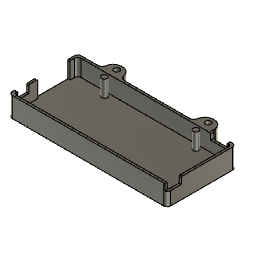
AramBadgeCase (Autodesk Fusion 360 design; units mm, degrees)
Autodesk Fusion 360 part; units mm, degrees
sketch "Sketch1" plane through (0, 0, 0) normal (0, 0, 1) x (1, 0, 0)
  line L0 (69.25, -29) -> (-69.25, -29)
  line L1 (-69.25, -29) -> (-69.25, 29)
  line L2 (-69.25, 29) -> (69.25, 29)
  line L3 (69.25, 29) -> (69.25, -29)
  line L4 (69.25, -29) -> (-69.25, 29) construction
  line L5 (-69.25, -29) -> (69.25, 29) construction
  line L6 (71.25, -31) -> (-71.25, -31)
  line L7 (-71.25, -31) -> (-71.25, 31)
  line L8 (-71.25, 31) -> (71.25, 31)
  line L9 (71.25, 31) -> (71.25, -31)
  line L10 (71.25, -31) -> (-71.25, 31) construction
  line L11 (-71.25, -31) -> (71.25, 31) construction
  dimension "d1" = 138.5
  dimension "d2" = 58
  dimension "d3" = 2
  dimension "d4" = 2
  constraint horizontal L0
  constraint perpendicular L0 L1
  constraint parallel L0 L2
  constraint parallel L1 L3
  constraint coincident L4 origin
  constraint coincident L5 origin
  constraint horizontal L6
  constraint perpendicular L6 L7
  constraint parallel L6 L8
  constraint parallel L7 L9
  constraint coincident L10 origin
  constraint coincident L11 origin
  measures "d1" distance of L1.end L2.end
  measures "d2" distance of L0.end L1.end
  measures "d3" distance of L1 L7
  measures "d4" distance of L2 L8
extrude "Extrude1" add sketch "Sketch1" along normal blind 15 makes body 1
sketch "Sketch3" plane through (0, 0, 15) normal (0, 0, 1) x (-1, 0, 0)
  line L0 (69.25, -29) -> (-69.25, -29)
  line L1 (-69.25, -29) -> (-69.25, 29)
  line L2 (-69.25, 29) -> (69.25, 29)
  line L3 (69.25, 29) -> (69.25, -29)
  line L4 (71.25, 31) -> (-71.25, 31)
  line L5 (-71.25, 31) -> (-71.25, -31)
  line L6 (-71.25, -31) -> (71.25, -31)
  line L7 (71.25, -31) -> (71.25, 31)
  line L8 (-65.25, -29) -> (-65.25, -31)
  line L9 (-50.25, -31) -> (-50.25, -29)
  line L10 (-69.25, 18) -> (-71.25, 18)
  line L11 (-71.25, 18) -> (-71.25, 31)
  line L12 (-71.25, 31) -> (-69.25, 31)
  line L13 (-69.25, 31) -> (-69.25, 18)
  line L14 (71.25, 15) -> (69.25, 15)
  line L15 (69.25, 25) -> (71.25, 25)
  dimension "d13" = 21
  dimension "d14" = 6
  dimension "d19" = 13
  dimension "d22" = 6
  dimension "d23" = 16
  constraint vertical L8
  constraint vertical L9
  constraint coincident L6 L8.end
  constraint coincident L0 L9.end
  constraint horizontal L10
  constraint vertical L11
  constraint horizontal L12
  constraint vertical L13
  constraint coincident L4.end L5.start
  constraint coincident L1 L10.start
  constraint horizontal L14
  constraint horizontal L15
  constraint coincident L3 L15.start
  constraint coincident L7 L14.start
  measures "d13" distance of L5.end L9
  measures "d14" distance of L5 L8
  measures "d19" distance of L10 L12
  measures "d22" distance of L4 L15.start
  measures "d23" distance of L4 L14.start
extrude "Extrude5" cut sketch "Sketch3" against normal blind 7 contours L3 L7 L14 L15 bodies 1
extrude "Extrude3" cut sketch "Sketch3" against normal blind 5.5 contours L0 L6 L8 L9 bodies 1
sketch "Sketch2" plane through (0, 0, 0) normal (0, 0, -1) x (1, 0, 0)
  line L0 (-71.25, 31) -> (-71.25, -31)
  line L1 (-71.25, -31) -> (71.25, -31)
  line L2 (71.25, -31) -> (71.25, 31)
  line L3 (71.25, 31) -> (-71.25, 31)
  line L4 (-69.25, -29) -> (-69.25, 29)
  line L5 (-69.25, 29) -> (69.25, 29)
  line L6 (69.25, 29) -> (69.25, -29)
  line L7 (69.25, -29) -> (-69.25, -29)
  circle A0 centre (41.25, -25) radius 2.5
  line L8 (-69.25, -29) -> (69.25, -29)
  line L9 (69.25, -29) -> (69.25, 29)
  dimension "d32" = 5
  dimension "d33" = 4
  dimension "d34" = 28
  measures "d32" diameter of A0
  measures "d33" distance of A0.centre L8
  measures "d34" distance of A0.centre L9
extrude "Extrude6" add sketch "Sketch2" against normal up to surface (15 mm away) separate body contours A0 makes body 2
extrude "Extrude2" add sketch "Sketch2" along normal blind 3 contours L0 L1 L2 L3 | L4 L5 L6 L7 L8 L9 | A0 bodies 1
extrude "Extrude4" cut sketch "Sketch3" against normal blind 6 contours L1 L4 L5 L10 L11 L12 L13 bodies 1
fillet "Fillet4" radius 3 4 edges at (71.25, -31, 3) (71.25, 31, 6) (-71.25, -31, 6) (-71.25, 31, 6) on bodies 1
fillet "Fillet5" radius 3 4 edges at (69.25, 29, 7.5) (-69.25, 29, 7.5) (-69.25, -29, 7.5) (69.25, -29, 4.5) on bodies 1
fillet "Fillet6" radius 1 5 edges at (-70.25, -15, 15) (-70.25, -25, 15) (65.25, 30, 15) (50.25, 30, 15) (70.25, -18, 15) on bodies 1
mirror "Mirror1" about plane through (0, 0, 0) normal (1, 0, 0) of bodies 2 makes body 3
sketch "Sketch4" plane through (0, 0, 15) normal (0, 0, 1) x (-1, 0, 0)
  line L0 (-49.25, -29) -> (-49.25, -31)
  line L1 (-49.25, -31) -> (68.25, -31)
  arc A0 (68.25, -31) -> (71.25, -28) centre (68.25, -28) ccw
  line L2 (71.25, -28) -> (71.25, 14)
  line L3 (71.25, 14) -> (69.25, 14)
  line L4 (69.25, 14) -> (69.25, -26)
  arc A1 (66.25, -29) -> (69.25, -26) centre (66.25, -26) ccw
  line L5 (66.25, -29) -> (-49.25, -29)
  line L6 (71.25, -22) -> (69.25, -22)
  line L7 (69.25, -22) -> (69.25, 7)
  line L8 (69.25, 7) -> (71.25, 7)
  line L9 (71.25, 7) -> (71.25, -22)
  line L10 (71.25, -31) -> (-71.25, -31)
  dimension "d39" = 9
  dimension "d40" = 38
  constraint horizontal L6
  constraint vertical L7
  constraint horizontal L8
  constraint vertical L9
  constraint coincident L4 L7.end
  constraint coincident L2 L6.start
  measures "d39" distance of L6 L10
  measures "d40" distance of L8 L10
extrude "Extrude7" cut sketch "Sketch4" against normal up to surface (15 mm away) contours L2 L4 L6 L7 L8 L9 bodies 1
fillet "Fillet7" radius 1 2 edges at (-70.25, 22, 15) (-70.25, -7, 15) on bodies 1
sketch "Sketch6" plane through (0, 31, 0) normal (0, 1, 0) x (-1, 0, 0)
  arc A0 (-49.25, 15) -> (-50.25, 14) centre (-49.25, 14) ccw
  line L0 (-50.25, 14) -> (-50.25, 9.5)
  line L1 (-50.25, 9.5) -> (-65.25, 9.5)
  line L2 (-65.25, 9.5) -> (-65.25, 14)
  arc A1 (-65.25, 14) -> (-66.25, 15) centre (-66.25, 14) ccw
  line L3 (-66.25, 15) -> (-68.25, 15)
  line L4 (-68.25, 15) -> (-68.25, -3)
  line L5 (-68.25, -3) -> (68.25, -3)
  line L6 (68.25, -3) -> (68.25, 15)
  line L7 (68.25, 15) -> (-49.25, 15)
  line L8 (-33.25, 15) -> (-49.25, 15)
  line L9 (-49.25, 15) -> (-49.25, -3)
  line L10 (-49.25, -3) -> (-33.25, -3)
  line L11 (-33.25, -3) -> (-33.25, 15)
  dimension "d47" = 19
  dimension "d48" = 16
  constraint horizontal L8
  constraint vertical L9
  constraint horizontal L10
  constraint vertical L11
  constraint coincident L5 L9.end
  constraint coincident L7 L8.start
  measures "d47" distance of L4 L9
  measures "d48" distance of L9 L11
extrude "Extrude9" add sketch "Sketch6" along normal blind 10 contours L5 L7 L8 L9 L10 L11 bodies 1
sketch "Sketch7" plane through (0, 0, 15) normal (0, 0, 1) x (-1, 0, 0)
  line L0 (71.25, -23) -> (69.25, -23)
  line L1 (69.25, -23) -> (69.25, -26)
  arc A0 (66.25, -29) -> (69.25, -26) centre (66.25, -26) ccw
  line L2 (66.25, -29) -> (-49.25, -29)
  line L3 (-49.25, -29) -> (-49.25, -31)
  line L4 (-49.25, -31) -> (-49.25, -41)
  line L5 (-49.25, -41) -> (-33.25, -41)
  line L6 (-33.25, -41) -> (-33.25, -31)
  line L7 (-33.25, -31) -> (68.25, -31)
  arc A1 (68.25, -31) -> (71.25, -28) centre (68.25, -28) ccw
  line L8 (71.25, -28) -> (71.25, -23)
  circle A2 centre (-41.25, -36) radius 2.5
  dimension "d51" = 5
  dimension "d52" = 8
  dimension "d53" = 5
  measures "d51" diameter of A2
  measures "d52" distance of L4 A2.centre
  measures "d53" distance of L5 A2.centre
extrude "Extrude10" cut sketch "Sketch7" against normal up to surface (18 mm away) contours A2 bodies 1
fillet "Fillet8" radius 7.5 2 edges at (49.25, 41, 6) (33.25, 41, 6) on bodies 1
mirror "Mirror2" about plane through (0, 0, 0) normal (1, 0, 0) of "Extrude9", "Extrude10", "Fillet8"
sketch "Sketch8" plane through (0, 0, -3) normal (0, 0, -1) x (1, 0, 0)
  circle A0 centre (-41.25, -36) radius 2.5
  arc A1 (-40.75, -41) -> (-33.25, -33.5) centre (-40.75, -33.5) ccw
  line L0 (-33.25, -33.5) -> (-33.25, -31)
  line L1 (-33.25, -31) -> (33.25, -31)
  line L2 (33.25, -31) -> (33.25, -33.5)
  arc A2 (33.25, -33.5) -> (40.75, -41) centre (40.75, -33.5) ccw
  line L3 (40.75, -41) -> (41.75, -41)
  arc A3 (41.75, -41) -> (49.25, -33.5) centre (41.75, -33.5) ccw
  line L4 (49.25, -33.5) -> (49.25, -31)
  line L5 (49.25, -31) -> (68.25, -31)
  arc A4 (68.25, -31) -> (71.25, -28) centre (68.25, -28) ccw
  line L6 (71.25, -28) -> (71.25, 28)
  arc A5 (71.25, 28) -> (68.25, 31) centre (68.25, 28) ccw
  line L7 (68.25, 31) -> (-68.25, 31)
  arc A6 (-68.25, 31) -> (-71.25, 28) centre (-68.25, 28) ccw
  line L8 (-71.25, 28) -> (-71.25, -28)
  arc A7 (-71.25, -28) -> (-68.25, -31) centre (-68.25, -28) ccw
  line L9 (-68.25, -31) -> (-49.25, -31)
  line L10 (-49.25, -31) -> (-49.25, -33.5)
  arc A8 (-49.25, -33.5) -> (-41.75, -41) centre (-41.75, -33.5) ccw
  line L11 (-41.75, -41) -> (-40.75, -41)
  circle A9 centre (41.25, -36) radius 2.5
  line L12 (-0.7094, -15.2047) -> (66.5141, -15.2047)
  line L13 (66.5141, -15.2047) -> (66.5141, 0.5508)
  line L14 (66.5141, 0.5508) -> (66.5141, 16.3063)
  line L15 (66.5141, 16.3063) -> (-0.7094, 16.3063)
  line L16 (-0.7094, 16.3063) -> (-67.9329, 16.3063)
  line L17 (-67.9329, 16.3063) -> (-67.9329, 0.5508)
  line L18 (-67.9329, 0.5508) -> (-67.9329, -15.2047)
  line L19 (-67.9329, -15.2047) -> (-0.7094, -15.2047)
  spline S0 degree 3 poles (-57.2192, 7.9034) (-55.8537, 7.9034) (-56.2739, 5.5926) (-58.1645, 3.4918) knots 0 0 0 0 1 1 1 1
  spline S1 degree 3 poles (-58.1645, 3.4918) (-59.7401, 1.7062) (-59.7401, 1.4961) (-57.9544, -0.4996) knots 0 0 0 0 1 1 1 1
  spline S2 degree 3 poles (-57.9544, -0.4996) (-54.9084, -3.8607) (-57.1141, -4.2809) (-60.5804, -1.0247) knots 0 0 0 0 1 1 1 1
  line L20 (-60.5804, -1.0247) -> (-63.7315, 2.0213)
  line L21 (-63.7315, 2.0213) -> (-60.8955, 4.9624)
  spline S3 degree 3 poles (-60.8955, 4.9624) (-59.3199, 6.5379) (-57.7444, 7.9034) (-57.2192, 7.9034) knots 0 0 0 0 1 1 1 1
  spline S4 degree 3 poles (-52.7026, 7.9034) (-51.5472, 7.9034) (-51.1271, 6.6429) (-51.1271, 2.6515) knots 0 0 0 0 1 1 1 1
  line L22 (-51.1271, 2.6515) -> (-51.1271, -2.6003)
  line L23 (-51.1271, -2.6003) -> (-47.4508, -2.6003)
  line L24 (-47.4508, -2.6003) -> (-43.7745, -2.6003)
  line L25 (-43.7745, -2.6003) -> (-43.7745, 2.6515)
  spline S5 degree 3 poles (-43.7745, 2.6515) (-43.7745, 6.6429) (-43.3543, 7.9034) (-42.1989, 7.9034) knots 0 0 0 0 1 1 1 1
  spline S6 degree 3 poles (-42.1989, 7.9034) (-40.9385, 7.9034) (-40.6234, 6.5379) (-40.6234, 2.1264) knots 0 0 0 0 1 1 1 1
  spline S7 degree 3 poles (-40.6234, 2.1264) (-40.6234, -4.0708) (-41.9889, -5.7514) (-47.4508, -5.7514) knots 0 0 0 0 1 1 1 1
  spline S8 degree 3 poles (-47.4508, -5.7514) (-52.9127, -5.7514) (-54.2782, -4.0708) (-54.2782, 2.1264) knots 0 0 0 0 1 1 1 1
  spline S9 degree 3 poles (-54.2782, 2.1264) (-54.2782, 6.5379) (-53.963, 7.9034) (-52.7026, 7.9034) knots 0 0 0 0 1 1 1 1
  spline S10 degree 3 poles (-37.2622, 6.6429) (-35.5816, 8.3235) (-27.8089, 8.3235) (-26.1283, 6.6429) knots 0 0 0 0 1 1 1 1
  spline S11 degree 3 poles (-26.1283, 6.6429) (-24.4477, 4.9624) (-24.6578, -2.3902) (-26.4434, -6.2766) knots 0 0 0 0 1 1 1 1
  spline S12 degree 3 poles (-26.4434, -6.2766) (-27.3887, -8.3773) (-27.9139, -8.7975) (-27.9139, -7.537) knots 0 0 0 0 1 1 1 1
  spline S13 degree 3 poles (-27.9139, -7.537) (-28.019, -6.1715) (-28.9643, -5.7514) (-31.6953, -5.7514) knots 0 0 0 0 1 1 1 1
  spline S14 degree 3 poles (-31.6953, -5.7514) (-34.4262, -5.7514) (-35.3715, -6.1715) (-35.4766, -7.537) knots 0 0 0 0 1 1 1 1
  spline S15 degree 3 poles (-35.4766, -7.537) (-35.4766, -8.7975) (-36.0018, -8.3773) (-36.9471, -6.2766) knots 0 0 0 0 1 1 1 1
  spline S16 degree 3 poles (-36.9471, -6.2766) (-38.7327, -2.3902) (-38.9428, 4.9624) (-37.2622, 6.6429) knots 0 0 0 0 1 1 1 1
  line L26 (-17.5153, -2.6003) -> (-12.2635, -2.6003)
  line L27 (-12.2635, -2.6003) -> (-12.2635, 1.076)
  line L28 (-12.2635, 1.076) -> (-12.2635, 4.7523)
  line L29 (-12.2635, 4.7523) -> (-17.5153, 4.7523)
  spline S17 degree 3 poles (-17.5153, 4.7523) (-21.5067, 4.7523) (-22.7671, 5.1724) (-22.7671, 6.3278) knots 0 0 0 0 1 1 1 1
  spline S18 degree 3 poles (-22.7671, 6.3278) (-22.7671, 8.3235) (-12.2635, 8.5336) (-10.3728, 6.6429) knots 0 0 0 0 1 1 1 1
  spline S19 degree 3 poles (-10.3728, 6.6429) (-9.6375, 5.9077) (-9.1124, 3.3868) (-9.1124, 0.8659) knots 0 0 0 0 1 1 1 1
  spline S20 degree 3 poles (-9.1124, 0.8659) (-9.1124, -4.491) (-10.898, -5.7514) (-17.9354, -5.7514) knots 0 0 0 0 1 1 1 1
  spline S21 degree 3 poles (-17.9354, -5.7514) (-21.5067, -5.7514) (-22.7671, -5.3312) (-22.7671, -4.1758) knots 0 0 0 0 1 1 1 1
  spline S22 degree 3 poles (-22.7671, -4.1758) (-22.7671, -3.0204) (-21.5067, -2.6003) (-17.5153, -2.6003) knots 0 0 0 0 1 1 1 1
  spline S23 degree 3 poles (-5.4361, 7.9034) (-4.2807, 7.9034) (-3.8605, 6.6429) (-3.8605, 2.6515) knots 0 0 0 0 1 1 1 1
  line L30 (-3.8605, 2.6515) -> (-3.8605, -2.6003)
  line L31 (-3.8605, -2.6003) -> (-0.1842, -2.6003)
  line L32 (-0.1842, -2.6003) -> (3.4921, -2.6003)
  line L33 (3.4921, -2.6003) -> (3.4921, 2.6515)
  spline S24 degree 3 poles (3.4921, 2.6515) (3.4921, 6.6429) (3.9122, 7.9034) (5.0676, 7.9034) knots 0 0 0 0 1 1 1 1
  spline S25 degree 3 poles (5.0676, 7.9034) (6.328, 7.9034) (6.6432, 6.5379) (6.6432, 2.1264) knots 0 0 0 0 1 1 1 1
  spline S26 degree 3 poles (6.6432, 2.1264) (6.6432, -4.0708) (5.2777, -5.7514) (-0.1842, -5.7514) knots 0 0 0 0 1 1 1 1
  spline S27 degree 3 poles (-0.1842, -5.7514) (-5.6461, -5.7514) (-7.0116, -4.0708) (-7.0116, 2.1264) knots 0 0 0 0 1 1 1 1
  spline S28 degree 3 poles (-7.0116, 2.1264) (-7.0116, 6.5379) (-6.6965, 7.9034) (-5.4361, 7.9034) knots 0 0 0 0 1 1 1 1
  spline S29 degree 3 poles (-0.1842, 7.9034) (0.9712, 7.9034) (1.3913, 6.6429) (1.3913, 3.1767) knots 0 0 0 0 1 1 1 1
  spline S30 degree 3 poles (1.3913, 3.1767) (1.3913, -0.2895) (0.9712, -1.5499) (-0.1842, -1.5499) knots 0 0 0 0 1 1 1 1
  spline S31 degree 3 poles (-0.1842, -1.5499) (-1.3396, -1.5499) (-1.7598, -0.2895) (-1.7598, 3.1767) knots 0 0 0 0 1 1 1 1
  spline S32 degree 3 poles (-1.7598, 3.1767) (-1.7598, 6.6429) (-1.3396, 7.9034) (-0.1842, 7.9034) knots 0 0 0 0 1 1 1 1
  spline S33 degree 3 poles (10.3194, 7.9034) (11.2648, 7.9034) (11.895, 6.9581) (11.895, 5.2775) knots 0 0 0 0 1 1 1 1
  spline S34 degree 3 poles (11.895, 5.2775) (11.895, 2.9667) (12.3151, 2.6515) (15.5713, 2.6515) knots 0 0 0 0 1 1 1 1
  spline S35 degree 3 poles (15.5713, 2.6515) (18.8274, 2.6515) (19.2476, 2.9667) (19.2476, 5.2775) knots 0 0 0 0 1 1 1 1
  spline S36 degree 3 poles (19.2476, 5.2775) (19.2476, 6.9581) (19.8778, 7.9034) (20.8231, 7.9034) knots 0 0 0 0 1 1 1 1
  spline S37 degree 3 poles (20.8231, 7.9034) (23.0289, 7.9034) (23.0289, -1.865) (20.7181, -4.0708) knots 0 0 0 0 1 1 1 1
  spline S38 degree 3 poles (20.7181, -4.0708) (18.8274, -5.9615) (13.7857, -6.2766) (10.7396, -4.701) knots 0 0 0 0 1 1 1 1
  spline S39 degree 3 poles (10.7396, -4.701) (9.164, -3.7557) (8.7439, -2.3902) (8.7439, 2.1264) knots 0 0 0 0 1 1 1 1
  spline S40 degree 3 poles (8.7439, 2.1264) (8.7439, 6.5379) (9.059, 7.9034) (10.3194, 7.9034) knots 0 0 0 0 1 1 1 1
  spline S41 degree 3 poles (29.9613, 2.4415) (34.4779, 2.7566) (35.0031, 2.9667) (35.0031, 5.3825) knots 0 0 0 0 1 1 1 1
  spline S42 degree 3 poles (35.0031, 5.3825) (35.0031, 6.9581) (35.6333, 7.9034) (36.5786, 7.9034) knots 0 0 0 0 1 1 1 1
  spline S43 degree 3 poles (36.5786, 7.9034) (37.8391, 7.9034) (38.1542, 6.4329) (38.1542, 1.076) knots 0 0 0 0 1 1 1 1
  line L34 (38.1542, 1.076) -> (38.1542, -5.7514)
  line L35 (38.1542, -5.7514) -> (32.5872, -5.7514)
  spline S44 degree 3 poles (32.5872, -5.7514) (26.285, -5.7514) (24.2893, -4.3859) (24.7095, -0.4996) knots 0 0 0 0 1 1 1 1
  spline S45 degree 3 poles (24.7095, -0.4996) (25.0246, 1.8113) (25.5498, 2.1264) (29.9613, 2.4415) knots 0 0 0 0 1 1 1 1
  spline S46 degree 3 poles (29.2261, 7.9034) (30.0664, 7.9034) (30.8016, 6.9581) (30.8016, 5.8026) knots 0 0 0 0 1 1 1 1
  spline S47 degree 3 poles (30.8016, 5.8026) (30.8016, 4.6472) (30.0664, 3.7019) (29.2261, 3.7019) knots 0 0 0 0 1 1 1 1
  spline S48 degree 3 poles (29.2261, 3.7019) (28.3858, 3.7019) (27.6505, 4.6472) (27.6505, 5.8026) knots 0 0 0 0 1 1 1 1
  spline S49 degree 3 poles (27.6505, 5.8026) (27.6505, 6.9581) (28.3858, 7.9034) (29.2261, 7.9034) knots 0 0 0 0 1 1 1 1
  spline S50 degree 3 poles (41.2002, 7.9034) (41.7254, 7.9034) (42.3557, 6.853) (42.5657, 5.5926) knots 0 0 0 0 1 1 1 1
  spline S51 degree 3 poles (42.5657, 5.5926) (42.7758, 3.5969) (43.6161, 3.0717) (46.7672, 2.8616) knots 0 0 0 0 1 1 1 1
  spline S52 degree 3 poles (46.7672, 2.8616) (50.4435, 2.5465) (50.7586, 2.7566) (50.7586, 5.1724) knots 0 0 0 0 1 1 1 1
  spline S53 degree 3 poles (50.7586, 5.1724) (50.7586, 6.853) (51.3888, 7.9034) (52.3341, 7.9034) knots 0 0 0 0 1 1 1 1
  spline S54 degree 3 poles (52.3341, 7.9034) (54.5399, 7.9034) (54.5399, -1.865) (52.2291, -4.0708) knots 0 0 0 0 1 1 1 1
  spline S55 degree 3 poles (52.2291, -4.0708) (50.3384, -5.9615) (45.2967, -6.2766) (42.2506, -4.701) knots 0 0 0 0 1 1 1 1
  spline S56 degree 3 poles (42.2506, -4.701) (40.6751, -3.7557) (40.2549, -2.3902) (40.2549, 2.1264) knots 0 0 0 0 1 1 1 1
  spline S57 degree 3 poles (40.2549, 2.1264) (40.2549, 5.2775) (40.6751, 7.9034) (41.2002, 7.9034) knots 0 0 0 0 1 1 1 1
  line L36 (58.1112, 0.0256) -> (60.2119, 2.3364)
  line L37 (60.2119, 2.3364) -> (58.1112, 4.2271)
  spline S58 degree 3 poles (58.1112, 4.2271) (56.9558, 5.2775) (56.0104, 6.5379) (56.0104, 7.0631) knots 0 0 0 0 1 1 1 1
  spline S59 degree 3 poles (56.0104, 7.0631) (56.0104, 8.8487) (58.8464, 7.7983) (61.5774, 4.9624) knots 0 0 0 0 1 1 1 1
  line L38 (61.5774, 4.9624) -> (64.4134, 2.0213)
  line L39 (64.4134, 2.0213) -> (61.4723, -0.8147)
  spline S60 degree 3 poles (61.4723, -0.8147) (56.8507, -5.2262) (53.9097, -4.491) (58.1112, 0.0256) knots 0 0 0 0 1 1 1 1
  spline S61 degree 3 poles (-31.6953, -2.6003) (-28.229, -2.6003) (-28.019, -2.3902) (-28.019, 1.076) knots 0 0 0 0 1 1 1 1
  spline S62 degree 3 poles (-28.019, 1.076) (-28.019, 4.5422) (-28.229, 4.7523) (-31.6953, 4.7523) knots 0 0 0 0 1 1 1 1
  spline S63 degree 3 poles (-31.6953, 4.7523) (-35.1615, 4.7523) (-35.3715, 4.5422) (-35.3715, 1.076) knots 0 0 0 0 1 1 1 1
  spline S64 degree 3 poles (-35.3715, 1.076) (-35.3715, -2.3902) (-35.1615, -2.6003) (-31.6953, -2.6003) knots 0 0 0 0 1 1 1 1
  spline S65 degree 3 poles (-33.2708, 0.5508) (-32.7456, 0.5508) (-32.2204, 0.1307) (-32.2204, -0.4996) knots 0 0 0 0 1 1 1 1
  spline S66 degree 3 poles (-32.2204, -0.4996) (-32.2204, -1.0247) (-32.7456, -1.5499) (-33.2708, -1.5499) knots 0 0 0 0 1 1 1 1
  spline S67 degree 3 poles (-33.2708, -1.5499) (-33.901, -1.5499) (-34.3212, -1.0247) (-34.3212, -0.4996) knots 0 0 0 0 1 1 1 1
  spline S68 degree 3 poles (-34.3212, -0.4996) (-34.3212, 0.1307) (-33.901, 0.5508) (-33.2708, 0.5508) knots 0 0 0 0 1 1 1 1
  spline S69 degree 3 poles (-30.1197, 0.5508) (-29.5945, 0.5508) (-29.0693, 0.1307) (-29.0693, -0.4996) knots 0 0 0 0 1 1 1 1
  spline S70 degree 3 poles (-29.0693, -0.4996) (-29.0693, -1.0247) (-29.5945, -1.5499) (-30.1197, -1.5499) knots 0 0 0 0 1 1 1 1
  spline S71 degree 3 poles (-30.1197, -1.5499) (-30.7499, -1.5499) (-31.1701, -1.0247) (-31.1701, -0.4996) knots 0 0 0 0 1 1 1 1
  spline S72 degree 3 poles (-31.1701, -0.4996) (-31.1701, 0.1307) (-30.7499, 0.5508) (-30.1197, 0.5508) knots 0 0 0 0 1 1 1 1
  spline S73 degree 3 poles (15.2562, -2.3902) (17.0418, -2.1801) (18.7224, -1.5499) (18.9325, -0.9197) knots 0 0 0 0 1 1 1 1
  spline S74 degree 3 poles (18.9325, -0.9197) (19.1425, -0.2895) (17.8821, -0.0794) (15.5713, -0.2895) knots 0 0 0 0 1 1 1 1
  spline S75 degree 3 poles (15.5713, -0.2895) (10.9497, -0.8147) (10.6346, -2.8104) (15.2562, -2.3902) knots 0 0 0 0 1 1 1 1
  spline S76 degree 3 poles (31.3268, -2.6003) (33.6376, -2.6003) (35.0031, -2.0751) (35.0031, -1.2348) knots 0 0 0 0 1 1 1 1
  spline S77 degree 3 poles (35.0031, -1.2348) (35.0031, -0.2895) (33.8477, 0.0256) (31.3268, -0.2895) knots 0 0 0 0 1 1 1 1
  spline S78 degree 3 poles (31.3268, -0.2895) (29.3311, -0.4996) (27.6505, -1.1298) (27.6505, -1.655) knots 0 0 0 0 1 1 1 1
  spline S79 degree 3 poles (27.6505, -1.655) (27.6505, -2.1801) (29.3311, -2.6003) (31.3268, -2.6003) knots 0 0 0 0 1 1 1 1
  spline S80 degree 3 poles (46.7672, -2.3902) (48.5528, -2.1801) (50.2334, -1.5499) (50.4435, -0.9197) knots 0 0 0 0 1 1 1 1
  spline S81 degree 3 poles (50.4435, -0.9197) (50.6536, -0.2895) (49.3931, -0.0794) (47.0823, -0.2895) knots 0 0 0 0 1 1 1 1
  spline S82 degree 3 poles (47.0823, -0.2895) (42.4607, -0.8147) (42.1456, -2.8104) (46.7672, -2.3902) knots 0 0 0 0 1 1 1 1
extrude "Extrude11" add sketch "Sketch8" along normal blind 0.5 contours S0 S1 S2 L20 L21 S3 | S4 L22 L23 L24 L25 S5 S6 S7 S8 S9 | S10 S11 S12 S13 S14 S15 S16 | L26 L27 L28 L29 S17 S18 S19 S20 S21 S22 | S23 L30 L31 L32 L33 S24 S25 S26 S27 S28 | S29 S30 S31 S32 | S33 S34 S35 S36 S37 S38 S39 S40 | S41 S42 S43 L34 L35 S44 S45 | S46 S47 S48 S49 | S50 S51 S52 S53 S54 S55 S56 S57 | L36 L37 S58 S59 L38 L39 S60 | S65 S66 S67 S68 | S69 S70 S71 S72 bodies 1
fillet "Fillet9" radius 4 4 edges at (-49.25, 31, 6) (-33.25, 31, 6) (49.25, 31, 6) (33.25, 31, 6) on bodies 1
